Right Angle Stepper Motor Mount_v6 (Autodesk Fusion 360 design; units mm, degrees)
Autodesk Fusion 360 part; units mm, degrees
note: some values were not read from the file. Set by a fixed rule: which sketch regions a step uses.
sketch "Sketch1" plane through (0, 0, 0) normal (0, 0, 1) x (1, 0, 0)
  line L0 (0, 0) -> (53, 0)
  line L1 (53, 0) -> (53, 50)
  line L2 (53, 50) -> (0, 50)
  line L3 (0, 50) -> (0, 0)
  line L4 (12, 7.9) -> (42, 7.9)
  arc A0 (42, 7.9) -> (42, 12.1) centre (42, 10) ccw
  line L5 (42, 12.1) -> (12, 12.1)
  arc A1 (12, 12.1) -> (12, 7.9) centre (12, 10) ccw
  line L6 (12, 10) -> (42, 10) construction
  line L7 (0, 25) -> (53, 25) construction
  line L8 (42, 37.9) -> (12, 37.9)
  arc A2 (12, 42.1) -> (12, 37.9) centre (12, 40) ccw
  line L9 (12, 42.1) -> (42, 42.1)
  arc A3 (42, 37.9) -> (42, 42.1) centre (42, 40) ccw
  line L10 (49.4724, 50) -> (53.0079, 46.4645)
  line L11 (49.4724, 50) -> (52.8478, 50) construction
  line L12 (49.4724, 0) -> (53.0079, 3.5355)
  line L13 (0, 50) -> (2, 50)
  line L14 (2, 50) -> (2, 0)
  line L15 (2, 0) -> (0, 0)
  line L16 (0, 0) -> (0, 50)
  dimension "d1" = 53
  dimension "d2" = 50
  dimension "d3" = 4.2
  dimension "d4" = 11
  dimension "d5" = 10
  dimension "d6" = 30
  dimension "d9" = 45
  dimension "d10" = 5
  constraint horizontal L0
  constraint vertical L1
  constraint horizontal L2
  constraint vertical L3
  constraint coincident L0.start L3.end
  constraint tangent L4 A0
  constraint tangent A0 L5
  constraint parallel L4 L5
  constraint tangent L5 A1
  constraint tangent L4 A1
  constraint horizontal L6
  constraint midpoint L3 L7.start
  constraint midpoint L1 L7.end
  constraint symmetric L4.start L7 A2.start
  constraint symmetric L4.end L7 L9.end
  constraint symmetric A0.end L7 L8.start
  constraint symmetric L5.end L7 L8.end
  constraint symmetric A0 L7 A3
  constraint symmetric A1 L7 A2
  constraint horizontal L11
  constraint coincident L2 L10.start
  constraint symmetric L7 L10.start L12.start
  constraint symmetric L7 L10.end L12.end
  constraint horizontal L13
  constraint vertical L14
  constraint horizontal L15
  constraint vertical L16
  constraint coincident L0 L14.end
  measures "d1" distance of L0.start L0.end
  measures "d2" distance of L0.start L2.end
  measures "d3" diameter of A0
  measures "d4" distance of L1 A0.centre
  measures "d5" distance of L0 L6
  measures "d6" distance of L4.start L4.end
  measures "d9" angle of L10 L11
  measures "d10" distance of L10.start L10.end
extrude "Extrude1" add sketch "Sketch1" against normal blind 2 contours L0 L2 L3 L13 L14 L15 L16 | L0 L1 L2 L10 L12 L14
extrude "Extrude2" add sketch "Sketch1" along normal blind 49 contours L0 L2 L3 L13 L14 L15 L16
sketch "Sketch2" plane through (0, 0, 0) normal (-1, 0, 0) x (0, -1, 0)
  line L0 (-50, 49) -> (-50, -2)
  line L1 (-50, -2) -> (0, -2)
  line L2 (0, -2) -> (0, 49)
  line L3 (0, 49) -> (-50, 49)
  circle A0 centre (-25, 23.5) radius 11.05
  line L4 (-40.5, 39) -> (-9.5, 39) construction
  line L5 (-9.5, 39) -> (-9.5, 8) construction
  line L6 (-9.5, 8) -> (-40.5, 8) construction
  line L7 (-40.5, 8) -> (-40.5, 39) construction
  line L8 (-40.5, 39) -> (-9.5, 8) construction
  line L9 (-9.5, 39) -> (-40.5, 8) construction
  circle A1 centre (-40.5, 39) radius 1.75
  circle A2 centre (-9.5, 39) radius 1.75
  circle A3 centre (-40.5, 8) radius 1.75
  circle A4 centre (-9.5, 8) radius 1.75
  line L10 (-50, 45.4997) -> (-46.4645, 49.0353)
  line L11 (-50, 45.4997) -> (-45, 45.4997) construction
  line L12 (-25, 49) -> (-25, -2)
  line L13 (0, 45.4997) -> (-3.5355, 49.0353)
  point P0 (-25, 23.5)
  dimension "d13" = 22.1
  dimension "d14" = 31
  dimension "d15" = 31
  dimension "d16" = 3.5
  dimension "d17" = 3.5
  dimension "d18" = 3.5
  dimension "d19" = 3.5
  dimension "d20" = 45
  dimension "d21" = 5
  constraint horizontal L4
  constraint perpendicular L4 L5
  constraint parallel L4 L6
  constraint parallel L5 L7
  constraint coincident L8 P0
  constraint coincident L9 P0
  constraint coincident P0 A0.centre
  constraint coincident L4.start L7.end
  constraint coincident L4.end L5.start
  constraint coincident L6.end L7.start
  constraint coincident L5.end L6.start
  constraint horizontal L11
  constraint coincident L0 L10.start
  constraint midpoint L3 L12.start
  constraint midpoint L1 L12.end
  constraint symmetric L10.start L12 L13.start
  constraint symmetric L10.end L12 L13.end
  measures "d13" diameter of A0
  measures "d14" distance of L5.end L6.end
  measures "d15" distance of L4.end L5.end
  measures "d16" diameter of A1
  measures "d17" diameter of A2
  measures "d18" diameter of A3
  measures "d19" diameter of A4
  measures "d20" angle of L10 L11
  measures "d21" distance of L10.start L10.end
extrude "Extrude3" cut sketch "Sketch2" against normal blind 2 contours L0 L3 L10 | L2 L3 L13 | A0 L12 | A0 L12 | A1 | A2 | A3 | A4
sketch "Sketch3" plane through (0, 0, 0) normal (0, -1, 0) x (1, 0, 0)
  line L0 (2, 45.4997) -> (0, 45.4997)
  line L1 (0, 45.4997) -> (0, -2)
  line L2 (0, -2) -> (49.4724, -2)
  line L3 (49.4724, -2) -> (49.4724, 0)
  line L4 (49.4724, 0) -> (2, 0)
  line L5 (2, 0) -> (2, 45.4997)
  line L6 (2, 0) -> (2, 20) construction
  line L7 (2, 0) -> (15, 0) construction
  line L8 (2, 20) -> (15, 0)
  dimension "d24" = 20
  dimension "d25" = 13
  constraint coincident L4.end L5.start
  constraint perpendicular L4 L6
  constraint perpendicular L5 L7
  measures "d24" distance of L4.end L6.end
  measures "d25" distance of L4.end L7.end
extrude "Extrude4" add sketch "Sketch3" against normal blind 2 contours L4 L5 L8
ref_plane "WorkPlane1" through (24.7362, 25, 21.7499) normal (0, -1, 0) x (-1, 0, 0)
mirror "Mirror1" about plane through (24.7362, 25, 21.7499) normal (0, -1, 0) of "Extrude4"
